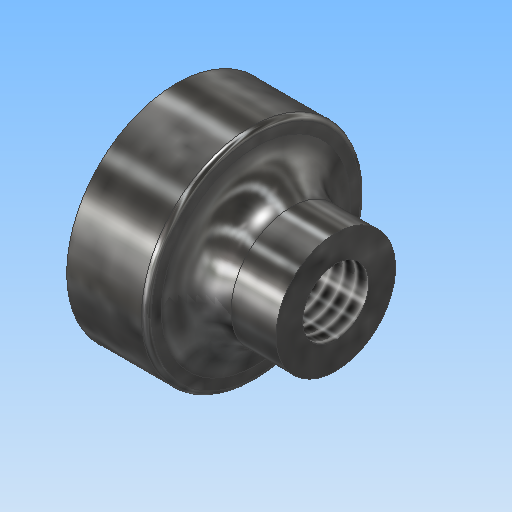
# Autodesk Inventor part: buje
Saved by Autodesk Inventor 2017 (Build 210142000, 142)
## iProperties
Part Number: buje
Material: Acero, alta resistencia, aleación baja
Document SubType Name: Modeling
Designer: Miguel A.
Density: 7.85 g/cm^3
Appearance: Acero galvanizado
Author: Miguel A.
Autodesk Inventor part; units mm, degrees
ref_plane "YZ Plane" through (0, 0, 0) normal (1, 0, 0) x (0, 1, 0)
ref_plane "XZ Plane" through (0, 0, 0) normal (0, 1, 0) x (-1, 0, 0)
ref_plane "XY Plane" through (0, 0, 0) normal (0, 0, 1) x (1, 0, 0)
sketch "cubrebola" plane through (0, 0, 0) normal (0, 0, 1) x (1, 0, 0)
  line L0 (-57.0337, 12.8146) -> (-57.0337, 11.8146)
  arc A0 (-57.0337, 11.8146) -> (-53.5337, 8.3146) centre (-53.5337, 11.8146) ccw
  line L1 (-53.5337, 8.3146) -> (-49.0337, 8.3146)
  line L2 (-49.0337, 8.3146) -> (-49.0337, 2.3146)
  line L3 (-57.5337, 13.3146) -> (-65.0337, 13.3146)
  line L4 (-65.0337, 13.3146) -> (-65.0337, 2.3146)
  line L5 (-65.0337, 2.3146) -> (-49.0337, 2.3146)
  line L6 (-53.2763, 2.3146) -> (-52.9205, 2.3146)
  arc A1 (-57.0337, 12.8146) -> (-57.5337, 13.3146) centre (-57.5337, 12.8146) ccw
  line L7 (-65.0337, 6.3146) -> (-49.0337, 6.3146) construction
  point P0 (-57.0337, 13.3146)
  dimension "d26" = 8
  dimension "d27" = 11
  dimension "d28" = 6
  dimension "d29" = 3.5
  dimension "d36" = 8
  dimension "d38" = 0.5
  dimension "d43" = 4
  dimension "d44" = 16
  dimension "d45" = 2
  measures "d26" distance of point (-57.034, 13.315) L3.end
  measures "d27" distance of L3.end L4.end
  measures "d28" distance of L1.end L2.end
  measures "d29" radius of A0
  measures "d36" distance from line of L2 point (-57.034, 13.315)
  measures "d38" radius of A1
  measures "d43" distance between parallel lines of L5 L7
  measures "d44" distance of L7.start L7.end
  measures "d45" distance between parallel lines of L7 L1
sketch "bola eje" plane through (0, 0, 0) normal (0, 0, 1) x (1, 0, 0)
  circle A0 centre (-63.7612, 5.5387) radius 3.5
  dimension "d25" = 3.5
  measures "d25" radius of A0
sketch "eje" plane through (0, 0, 0) normal (0, 0, 1) x (1, 0, 0)
  line L0 (-50.226, 18.6479) -> (-45.226, 18.6479)
  line L1 (-45.226, 18.6479) -> (-40.226, 16.6479)
  line L2 (-48.726, 4.3979) -> (-1.726, 4.3979)
  line L3 (-1.726, 4.3979) -> (-1.726, 16.6479)
  line L4 (-55.726, 11.1479) -> (-55.726, 16.1479)
  line L5 (-55.726, 16.1479) -> (-53.226, 18.6479)
  line L6 (-53.226, 18.6479) -> (-53.226, 27.1479)
  arc A0 (-50.226, 27.1479) -> (-53.226, 27.1479) centre (-51.726, 27.1479) ccw
  line L7 (-50.226, 27.1479) -> (-50.226, 18.6479)
  line L8 (-40.226, 16.6479) -> (-1.726, 16.6479)
  line L9 (-55.726, 11.1479) -> (-52.226, 11.1479)
  arc A1 (-48.726, 7.6479) -> (-52.226, 11.1479) centre (-52.226, 7.6479) ccw
  line L10 (-48.726, 7.6479) -> (-48.726, 4.3979)
  line L11 (-85.079, -1.8521) -> (81.6269, -1.8521) construction
  point P0 (0, 0)
  point P1 (-47.726, 18.6479)
  point P2 (-1.726, 10.5229)
  point P3 (-1.726, -1.8521)
  dimension "d15" = 12.5
  dimension "d47" = 3
  dimension "d48" = 135
  dimension "d49" = 4
  dimension "d50" = 7
  dimension "d51" = 3.5
  dimension "d52" = 5
  dimension "d53" = 12
  dimension "d54" = 2
  dimension "d55" = 5
  dimension "d56" = 5
  dimension "d57" = 12.25
  dimension "d58" = 6.75
  dimension "d59" = 10
  dimension "d62" = 50
  measures "d15" diameter of L2 L11
  measures "d47" distance between parallel lines of L6 L7
  measures "d48" angle of L4 L5
  measures "d49" horizontal distance of L4.end A0.centre
  measures "d50" distance between parallel lines of L10 L4
  measures "d51" radius of A1
  measures "d52" distance of L4.start L4.end
  measures "d54" distance between parallel lines of L8 L0
  measures "d55" distance of L0.start L0.end
  measures "d56" horizontal distance of L1.end L0.end
  measures "d57" distance between parallel lines of L8 L2
  measures "d58" distance between parallel lines of L2 L9
  measures "d62" distance from line of A0.centre L3
sketch "llanta" plane through (0, 0, 0) normal (0, 0, 1) x (1, 0, 0)
  arc A0 (-5.0239, 188.8921) -> (0, 187.1179) centre (0, 195.1179) ccw
  arc A1 (-16.5, 226.1566) -> (-16.5, 228.1566) centre (-16.5, 227.1566) ccw
  line L0 (-17.5, 228.1566) -> (-16.5, 228.1566)
  arc A2 (-17.5, 228.1566) -> (-18.5, 227.1566) centre (-17.5, 227.1566) ccw
  line L1 (-18.5, 227.1566) -> (-18.5, 202.1566)
  arc A3 (-18.5, 202.1566) -> (-16.6399, 198.2655) centre (-13.5, 202.1566) ccw
  line L2 (-16.6399, 198.2655) -> (-5.0239, 188.8921)
  arc A4 (-5.0239, 188.8921) -> (0, 187.1179) centre (0, 195.1179) ccw
  line L3 (-16.5, 226.1566) -> (-16.5, 202.1566)
  arc A5 (-16.5, 202.1566) -> (-15.3839, 199.822) centre (-13.5, 202.1566) ccw
  line L4 (-15.3839, 199.822) -> (-3.7679, 190.4485)
  arc A6 (-3.7679, 190.4485) -> (0, 189.1179) centre (0, 195.1179) ccw
  line L5 (0, 187.1179) -> (0, 189.1179)
  line L6 (0, 188.1179) -> (0, 205.2521) construction
  line L7 (15.3839, 199.822) -> (3.7679, 190.4485)
  line L8 (16.6399, 198.2655) -> (5.0239, 188.8921)
  arc A7 (0, 189.1179) -> (3.7679, 190.4485) centre (0, 195.1179) ccw
  arc A8 (0, 187.1179) -> (5.0239, 188.8921) centre (0, 195.1179) ccw
  arc A9 (0, 187.1179) -> (5.0239, 188.8921) centre (0, 195.1179) ccw
  arc A10 (15.3839, 199.822) -> (16.5, 202.1566) centre (13.5, 202.1566) ccw
  arc A11 (16.6399, 198.2655) -> (18.5, 202.1566) centre (13.5, 202.1566) ccw
  line L9 (16.5, 226.1566) -> (16.5, 202.1566)
  line L10 (18.5, 227.1566) -> (18.5, 202.1566)
  arc A12 (16.5, 228.1566) -> (16.5, 226.1566) centre (16.5, 227.1566) ccw
  line L11 (17.5, 228.1566) -> (16.5, 228.1566)
  arc A13 (18.5, 227.1566) -> (17.5, 228.1566) centre (17.5, 227.1566) ccw
  point P0 (-50.5, 240.1608)
  dimension "d63" = 2
  dimension "d65" = 25
  dimension "d66" = 5
  dimension "d67" = 8
  dimension "d69" = 2
  measures "d63" distance between parallel lines of L1 L3
  measures "d65" vertical distance of A2.centre A3.centre
  measures "d66" radius of A3
  measures "d67" radius of A4
  measures "d69" diameter of A1
derived "madre boceto.ipt"
sketch "Boceto1" plane through (0, 0, 0) normal (0, 0, 1) x (1, 0, 0)
  line L0 (0, 378.1944) -> (0, -378.1944)
  line L1 (-78.3437, 0) -> (85.8171, 0)
  circle A0 centre (-50.5, 9.5) radius 3.5
  line L2 (-54, 10.5) -> (-54, 9.5)
  arc A1 (-54, 9.5) -> (-50.5, 6) centre (-50.5, 9.5) ccw
  line L3 (-50.5, 6) -> (-46, 6)
  line L4 (-46, 6) -> (-46, 0)
  line L5 (-54.5, 11) -> (-62, 11)
  line L6 (-62, 11) -> (-62, 0)
  line L7 (-62, 0) -> (-46, 0)
  line L8 (-50.2426, 0) -> (-49.8867, 0)
  arc A2 (-54, 10.5) -> (-54.5, 11) centre (-54.5, 10.5) ccw
  line L9 (-62, 4) -> (-46, 4) construction
  line L10 (-48.5, 20.5) -> (-43.5, 20.5)
  line L11 (-43.5, 20.5) -> (-38.5, 18.5)
  line L12 (-47, 6.25) -> (0, 6.25)
  line L13 (0, 6.25) -> (0, 18.5)
  line L14 (-54, 13) -> (-54, 18)
  line L15 (-54, 18) -> (-51.5, 20.5)
  line L16 (-51.5, 20.5) -> (-51.5, 29)
  arc A3 (-48.5, 29) -> (-51.5, 29) centre (-50, 29) ccw
  line L17 (-48.5, 29) -> (-48.5, 20.5)
  line L18 (-38.5, 18.5) -> (0, 18.5)
  line L19 (-54, 13) -> (-50.5, 13)
  arc A4 (-47, 9.5) -> (-50.5, 13) centre (-50.5, 9.5) ccw
  line L20 (-47, 9.5) -> (-47, 6.25)
  line L21 (-83.3529, 0) -> (83.3529, 0) construction
  arc A5 (-5.0239, 401.7742) -> (0, 400) centre (0, 408) ccw
  arc A6 (-16.5, 439.0388) -> (-16.5, 441.0388) centre (-16.5, 440.0388) ccw
  line L22 (-17.5, 441.0388) -> (-16.5, 441.0388)
  arc A7 (-17.5, 441.0388) -> (-18.5, 440.0388) centre (-17.5, 440.0388) ccw
  line L23 (-18.5, 440.0388) -> (-18.5, 415.0388)
  arc A8 (-18.5, 415.0388) -> (-16.6399, 411.1476) centre (-13.5, 415.0388) ccw
  line L24 (-16.6399, 411.1476) -> (-5.0239, 401.7742)
  arc A9 (-5.0239, 401.7742) -> (0, 400) centre (0, 408) ccw
  line L25 (-16.5, 439.0388) -> (-16.5, 415.0388)
  arc A10 (-16.5, 415.0388) -> (-15.3839, 412.7041) centre (-13.5, 415.0388) ccw
  line L26 (-15.3839, 412.7041) -> (-3.7679, 403.3306)
  arc A11 (-3.7679, 403.3306) -> (0, 402) centre (0, 408) ccw
  line L27 (0, 400) -> (0, 402)
  line L28 (0, 401) -> (0, 418.1342) construction
  line L29 (15.3839, 412.7041) -> (3.7679, 403.3306)
  line L30 (16.6399, 411.1476) -> (5.0239, 401.7742)
  arc A12 (0, 402) -> (3.7679, 403.3306) centre (0, 408) ccw
  arc A13 (0, 400) -> (5.0239, 401.7742) centre (0, 408) ccw
  arc A14 (0, 400) -> (5.0239, 401.7742) centre (0, 408) ccw
  arc A15 (15.3839, 412.7041) -> (16.5, 415.0388) centre (13.5, 415.0388) ccw
  arc A16 (16.6399, 411.1476) -> (18.5, 415.0388) centre (13.5, 415.0388) ccw
  line L31 (16.5, 439.0388) -> (16.5, 415.0388)
  line L32 (18.5, 440.0388) -> (18.5, 415.0388)
  arc A17 (16.5, 441.0388) -> (16.5, 439.0388) centre (16.5, 440.0388) ccw
  line L33 (17.5, 441.0388) -> (16.5, 441.0388)
  arc A18 (18.5, 440.0388) -> (17.5, 441.0388) centre (17.5, 440.0388) ccw
  point P0 (0, 0)
  point P1 (0, 0)
revolve "Revolución1" add sketch "Boceto1" angle 360 about axis through (-83.3529, 0, 0) along (1, 0, 0) contours L1 L6 L5 A2 L2 A0 L3 L4
hole "Agujero1" at (-62, 0, 0) direction (1, 0, 0) diameter 6.647 depth 22.2 tip angle 118 thread size "M8x1.25" class "6H" standard "ISO Metric profile"
